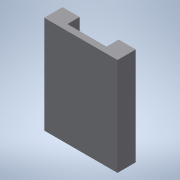
# Autodesk Inventor part: SP51V1 Cuerpo Freno
Saved by Autodesk Inventor 2021.2 (Build 252289000, 289)
## iProperties
Created: 2026-09-07
Part Number: SP51V1 Cuerpo Freno
Material: Generic
Document SubType Name: Modeling
Designer: nelso
Density: 1 g/cm^3
Appearance: Default
Author: nelso
Autodesk Inventor part; units mm, degrees
ref_plane "YZ Plane" through (0, 0, 0) normal (1, 0, 0) x (0, 1, 0)
ref_plane "XZ Plane" through (0, 0, 0) normal (0, 1, 0) x (-1, 0, 0)
ref_plane "XY Plane" through (0, 0, 0) normal (0, 0, 1) x (1, 0, 0)
sketch "Sketch1" plane through (0, 0, 0) normal (0, 1, 0) x (-1, 0, 0)
  line L0 (30, 40) -> (-30, 40)
  line L1 (-30, 40) -> (-30, -40)
  line L2 (-30, -40) -> (30, -40)
  line L3 (30, -40) -> (30, 40)
  line L4 (30, 40) -> (-30, -40) construction
  line L5 (-30, 40) -> (30, -40) construction
  point P0 (0, 0)
  dimension "d0" = 60
  dimension "d1" = 80
  constraints: 12 end point, 2 midpoint, 2 parallel, 1 horizontal, 1 perpendicular
  measures "d0" distance of L2.end L1.end
  measures "d1" distance of L1.end L0.end
extrude "Extrusion1" add sketch "Sketch1" along normal blind 15
sketch "Sketch2" plane through (0, 15, 0) normal (0, 1, 0) x (1, 0, 0)
  line L0 (30, 40) -> (-30, 40) projected
  line L1 (0, 40) -> (16, 40)
  line L2 (-30, -40) -> (30, -40) projected
  line L3 (16, 40) -> (-16, 40)
  line L4 (-16, 40) -> (-16, -40)
  line L5 (-16, -40) -> (16, -40)
  line L6 (16, -40) -> (16, 40)
  point P0 (0, 0)
  dimension "d4" = 16
  dimension "d5" = 32
  constraints: 10 end point, 2 parallel, 2 point on line, 1 horizontal, 1 midpoint, 1 perpendicular
  measures "d4" distance of L1.start L1.end
  measures "d5" distance of L5.end L4.end
extrude "Extrusion2" cut sketch "Sketch2" against normal blind 10
body "Solid1"
